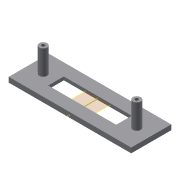
# Autodesk Inventor part: Top 6_7
Saved by Autodesk Inventor 2016 (Build 200138000, 138)
## iProperties
Created: 2015-04-13
Part Number: Top 6_7
Material: Generic
Document SubType Name: Modeling
Designer: Jonathan
Density: 1 g/cm^3
Appearance: Default
Mass: 13.6912 g
Surface Area: 101.938 cm^2
Volume: 13.6912 cm^3
Author: Jonathan
Autodesk Inventor part; units mm, degrees
ref_plane "YZ Plane" through (0, 0, 0) normal (1, 0, 0) x (0, 1, 0)
ref_plane "XZ Plane" through (0, 0, 0) normal (0, 1, 0) x (-1, 0, 0)
ref_plane "XY Plane" through (0, 0, 0) normal (0, 0, 1) x (1, 0, 0)
sketch "Sketch1" plane through (0, 0, 0) normal (0, 1, 0) x (-1, 0, 0)
  line L0 (55, -18) -> (-55, -18)
  line L1 (-55, -18) -> (-55, 18)
  line L2 (-55, 18) -> (55, 18)
  line L3 (55, 18) -> (55, -18)
  line L4 (55, -18) -> (-55, 18) construction
  line L5 (-55, -18) -> (55, 18) construction
  point P0 (0, 0)
  dimension "d0" = 110
  dimension "d1" = 36
  constraints: 12 end point, 2 midpoint, 2 parallel, 1 horizontal, 1 perpendicular
  measures "d0" distance of L1.end L2.end
  measures "d1" distance of L0.end L1.end
extrude "Body" add sketch "Sketch1" along normal mid plane 4.5
ref_plane "Work Plane4" through (0, 0.75, 0) normal (0, 1, 0) x (1, 0, 0)
sketch "Sketch6" plane through (0, 0.75, 0) normal (0, 1, 0) x (1, 0, 0)
  line L0 (-30.5, 7) -> (30.5, 7)
  line L1 (30.5, 7) -> (30.5, -7)
  line L2 (30.5, -7) -> (-30.5, -7)
  line L3 (-30.5, -7) -> (-30.5, 7)
  line L4 (-30.5, 7) -> (30.5, -7) construction
  line L5 (30.5, 7) -> (-30.5, -7) construction
  point P0 (0, 0)
  dimension "d15" = 61
  dimension "d16" = 14
  constraints: 12 end point, 2 midpoint, 2 parallel, 1 horizontal, 1 perpendicular
  measures "d15" distance of L1.end L2.end
  measures "d16" distance of L0.end L1.end
extrude "Flow Volume" cut sketch "Sketch6" along normal through all both and the other way through all
sketch "Sketch14" plane through (0, 2.25, 0) normal (0, 1, 0) x (1, 0, 0)
  line L0 (38.5, 18) -> (38.5, -18) projected
  line L1 (38.5, 0) -> (55, 0)
  line L2 (55, 18) -> (55, -18) projected
  circle A0 centre (42, 0) radius 3.5
  point P0 (0, 0)
  dimension "d37" = 7
  constraints: 2 end point, 2 midpoint, 1 horizontal alignment, 1 point on line, 2 other
extrude "Inlet" add sketch "Sketch14" along normal blind 22
sketch "Sketch15" plane through (42, 24.25, 0) normal (0, 1, 0) x (1, 0, 0)
  circle A0 centre (0, 0) radius 1.5
  circle A1 centre (0, 0) radius 3.5 projected
  point P0 (-42, 0)
  dimension "d40" = 3
  constraints: 1 centre point, 1 concentric
  measures "d40" diameter of A0
extrude "Inlet Hole" cut sketch "Sketch15" against normal through all contours A0
ref_plane "Work Plane1" through (0, 0.75, 18) normal (-1, 0, 0) x (0, 0, -1)
mirror "Outlet" about plane through (0, 0.75, 18) normal (-1, 0, 0) of "Inlet", "Inlet Hole"
sketch "Sketch22" plane through (0, -2.25, 0) normal (0, -1, 0) x (1, 0, 0)
  line L0 (-42.5, -13) -> (42.5, -13)
  line L1 (47.5, -8) -> (47.5, 8)
  line L2 (42.5, 13) -> (-42.5, 13)
  line L3 (-47.5, 8) -> (-47.5, -8)
  line L4 (-47.5, -13) -> (47.5, 13) construction
  line L5 (47.5, -13) -> (-47.5, 13) construction
  line L6 (-42.5, -13.5) -> (42.5, -13.5)
  line L7 (48, -8) -> (48, 8)
  line L8 (42.5, 13.5) -> (-42.5, 13.5)
  line L9 (-48, 8) -> (-48, -8)
  line L10 (-48, -13.5) -> (48, 13.5) construction
  line L11 (48, -13.5) -> (-48, 13.5) construction
  arc A0 (-47.5, -8) -> (-42.5, -13) centre (-42.5, -8) ccw
  arc A1 (42.5, -13) -> (47.5, -8) centre (42.5, -8) ccw
  arc A2 (47.5, 8) -> (42.5, 13) centre (42.5, 8) ccw
  arc A3 (-42.5, 13) -> (-47.5, 8) centre (-42.5, 8) ccw
  arc A4 (-48, -8) -> (-42.5, -13.5) centre (-42.5, -8) ccw
  arc A5 (42.5, -13.5) -> (48, -8) centre (42.5, -8) ccw
  arc A6 (48, 8) -> (42.5, 13.5) centre (42.5, 8) ccw
  arc A7 (-42.5, 13.5) -> (-48, 8) centre (-42.5, 8) ccw
  point P0 (0, 0)
  dimension "d56" = 95
  dimension "d57" = 26
  dimension "d58" = 0.5
  dimension "d59" = 0.5
  dimension "d60" = 5
  dimension "d61" = 5.5
  constraints: 24 end point, 16 point on circle, 16 point on line, 16 tangent, 8 centre point, 6 equal radius, 4 midpoint, 4 parallel, 2 horizontal, 2 perpendicular
  measures "d56" distance of L5.end L4.end
  measures "d57" distance of L5.end L4.start
  measures "d58" distance between parallel lines of L8 L2
  measures "d59" distance between parallel lines of L9 L3
  measures "d60" radius of A0
  measures "d61" radius of A4
extrude "Knife Edge" add sketch "Sketch22" along normal blind 1
sketch "Sketch23" plane through (0, -2.25, 0) normal (0, -1, 0) x (1, 0, 0)
  line L0 (38.5, 13) -> (-38.5, 13)
  line L1 (-38.5, 13) -> (-38.5, -13)
  line L2 (-38.5, -13) -> (38.5, -13)
  line L3 (38.5, -13) -> (38.5, 13)
  line L4 (38.5, 13) -> (-38.5, -13) construction
  line L5 (-38.5, 13) -> (38.5, -13) construction
  line L6 (-42.5, -13) -> (42.5, -13) projected
  point P0 (0, 0)
  dimension "d64" = 77
  constraints: 12 end point, 2 midpoint, 2 parallel, 1 collinear, 1 horizontal, 1 perpendicular
  measures "d64" distance of L2.end L1.end
extrude "Extrusion14" cut sketch "Sketch23" against normal blind 1.5
body "Solid1"
